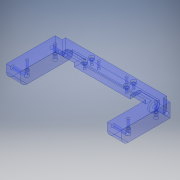
# Autodesk Inventor part: ElevBase
Saved by Autodesk Inventor 2019 (Build 230136000, 136)
## iProperties
Created: 2019-10-03
Part Number: ElevBase
Material: Generic
Document SubType Name: Modeling
Designer: james
Density: 1 g/cm^3
Appearance: Clear - Blue
Author: james
Autodesk Inventor part; units mm, degrees
ref_plane "YZ Plane" through (0, 0, 0) normal (1, 0, 0) x (0, 1, 0)
ref_plane "XZ Plane" through (0, 0, 0) normal (0, 1, 0) x (-1, 0, 0)
ref_plane "XY Plane" through (0, 0, 0) normal (0, 0, 1) x (1, 0, 0)
sketch "Sketch1" plane through (0, 0, 0) normal (0, 1, 0) x (-1, 0, 0)
  line L0 (153.7387, 43.057) -> (128.3387, 43.057)
  line L1 (128.3387, 43.057) -> (128.3387, -26.793)
  line L2 (128.3387, -26.793) -> (-30.4113, -26.793)
  line L3 (-30.4113, -26.793) -> (-30.4113, 43.057)
  line L4 (-30.4113, 43.057) -> (-55.8113, 43.057)
  line L5 (-55.8113, 43.057) -> (-55.8113, -52.193)
  line L6 (-55.8113, -52.193) -> (153.7387, -52.193)
  line L7 (153.7387, -52.193) -> (153.7387, 43.057)
  point P0 (0, 0)
  dimension "d0" = 95.25
  dimension "d1" = 25.4
  dimension "d2" = 25.4
  dimension "d3" = 158.75
  dimension "d4" = 25.4
  constraints: 16 end point, 6 perpendicular, 3 point on line, 1 horizontal
  measures "d0" distance of L6.end L0.start
  measures "d1" distance between parallel lines of L1 L7
  measures "d2" distance between parallel lines of L5 L3
  measures "d3" distance between parallel lines of L1 L3
  measures "d4" distance between parallel lines of L2 L6
extrude "Extrusion1" add sketch "Sketch1" along normal blind 25.4
sketch "Sketch2" plane through (55.8113, 0, 43.057) normal (1, 0, 0) x (0, 0, -1)
  line L0 (0, 0) -> (0, 25.4) projected
  line L1 (0, 0) -> (95.25, 0) projected
  point P0 (43.057, 0)
  point P1 (10.16, 15.24)
  dimension "d7" = 10.16
  dimension "d8" = 15.24
  measures "d7" distance from line of L0 point (10.16, 15.24)
  measures "d8" distance from line of L1 point (10.16, 15.24)
hole "Hole1" at (55.8113, 15.24, 32.897) direction (-1, 0, 0) diameter 6.477 end through all
fillet "Fillet2" radius 12.7 2 edges at (-141.0387, 0, 43.057) (43.1113, 0, 43.057)
sketch "Sketch3" plane through (0, 25.4, 0) normal (0, 1, 0) x (1, 0, 0)
  line L0 (-153.7387, 52.193) -> (-153.7387, -43.057) projected
  line L1 (55.8113, 52.193) -> (-153.7387, 52.193) projected
  line L2 (-128.3387, 26.793) -> (30.4113, 26.793) projected
  line L3 (55.8113, -43.057) -> (55.8113, 52.193) projected
  point P0 (0, 0)
  point P1 (-87.0637, 45.843)
  point P2 (-87.0637, 33.143)
  point P3 (-10.8637, 45.843)
  point P4 (-10.8637, 33.143)
  dimension "d19" = 66.675
  dimension "d20" = 6.35
  dimension "d21" = 0
  dimension "d22" = 6.35
  dimension "d23" = 0
  dimension "d24" = 6.35
  dimension "d25" = 6.35
  dimension "d26" = 66.675
  dimension "d64" = 76.2
  measures "d19" distance from line of L0 point (-87.064, 45.843)
  measures "d20" distance from line of L1 point (-87.064, 45.843)
  measures "d21" horizontal distance of point (-87.064, 45.843) point (-87.064, 33.143)
  measures "d22" distance from line of L2 point (-87.064, 33.143)
  measures "d23" horizontal distance of point (-10.864, 33.143) point (-10.864, 45.843)
  measures "d24" distance from line of L1 point (-10.864, 45.843)
  measures "d25" distance from line of L2 point (-10.864, 33.143)
  measures "d26" distance from line of L3 point (-10.864, 33.143)
  measures "d64" distance of point (-10.864, 45.843) point (-87.064, 45.843)
hole "Hole2" at (-87.0637, 25.4, -45.843) at (-87.0637, 25.4, -33.143) at (-10.8637, 25.4, -45.843) at (-10.8637, 25.4, -33.143) direction (0, -1, 0) diameter 4.4958 end through all counterbore diameter 7.9502 counterbore depth 4.1656 clearance for "Socket Head Cap Screw" size "#8" standard "Ansi Unified Screw Threads"
sketch "Sketch5" plane through (0, 0, 0) normal (0, -1, 0) x (1, 0, 0)
  line L0 (55.8113, -52.193) -> (-153.7387, -52.193) projected
  line L1 (55.8113, 43.057) -> (55.8113, -52.193) projected
  line L2 (-153.7387, -52.193) -> (-153.7387, 43.057) projected
  point P0 (0, 0)
  point P1 (-141.0387, -33.143)
  point P2 (-141.0387, 17.657)
  point P3 (43.1113, -33.143)
  point P4 (43.1113, 17.657)
  dimension "d34" = 19.05
  dimension "d35" = 12.7
  dimension "d36" = 12.7
  dimension "d37" = 50.8
  dimension "d38" = 12.7
  dimension "d39" = 19.05
  dimension "d40" = 12.7
  dimension "d41" = 50.8
  measures "d34" distance from line of L0 point (43.111, -33.143)
  measures "d35" distance from line of L1 point (43.111, -33.143)
  measures "d36" distance from line of L1 point (43.111, 17.657)
  measures "d37" distance of point (43.111, 17.657) point (43.111, -33.143)
  measures "d38" distance from line of L2 point (-141.039, -33.143)
  measures "d39" distance from line of L0 point (-141.039, -33.143)
  measures "d40" distance from line of L2 point (-141.039, 17.657)
  measures "d41" distance of point (-141.039, -33.143) point (-141.039, 17.657)
hole "Hole3" at (-141.0387, 0, -33.143) at (-141.0387, 0, 17.657) at (43.1113, 0, -33.143) at (43.1113, 0, 17.657) direction (0, 1, 0) diameter 4.4958 end through all clearance for "Socket Head Cap Screw" size "#8" standard "Ansi Unified Screw Threads"
sketch "Sketch6" plane through (0, 0, 0) normal (0, -1, 0) x (1, 0, 0)
  circle A0 centre (43.1113, -33.143) radius 2.2479 projected
  circle A1 centre (43.1113, 17.657) radius 2.2479 projected
  circle A2 centre (-141.0387, 17.657) radius 2.2479 projected
  circle A3 centre (-141.0387, -33.143) radius 2.2479 projected
  circle A4 centre (-141.0387, -33.143) radius 3.3734
  circle A5 centre (43.1113, -33.143) radius 3.3734
  circle A6 centre (43.1113, 17.657) radius 3.3734
  circle A7 centre (-141.0387, 17.657) radius 3.3734
  point P0 (0, 0)
  dimension "d49" = 6.7469
  dimension "d50" = 6.7469
  dimension "d51" = 6.7469
  dimension "d52" = 6.7469
  constraints: 4 centre point, 4 coincident
  measures "d49" diameter of A4
  measures "d50" diameter of A5
  measures "d51" diameter of A6
  measures "d52" diameter of A7
extrude "Extrusion2" cut sketch "Sketch6" against normal blind 9.525 contours A0 | A1 | A2 | A3 | A4 | A5 | A6 | A7
sketch "Sketch7" plane through (55.8113, 0, -52.193) normal (1, 0, 0) x (0, 0, -1)
  line L0 (0, 0) -> (0, 25.4) projected
  line L1 (-95.25, 25.4) -> (0, 25.4) projected
  point P0 (-52.193, 0)
  point P1 (-12.7, 10.16)
  dimension "d55" = 12.7
  dimension "d56" = 15.24
  measures "d55" distance from line of L0 point (-12.7, 10.16)
  measures "d56" distance from line of L1 point (-12.7, 10.16)
hole "Hole4" at (55.8113, 10.16, -39.493) direction (-1, 0, 0) diameter 6.477 end through all
sketch "Sketch8" plane through (0, 0, 0) normal (0, -1, 0) x (1, 0, 0)
  line L0 (1.8363, -26.793) -> (30.4113, -26.793)
  line L1 (30.4113, -26.793) -> (30.4113, -52.193)
  line L2 (30.4113, -52.193) -> (1.8363, -52.193)
  line L3 (1.8363, -52.193) -> (1.8363, -26.793)
  line L4 (30.4113, -26.793) -> (30.4113, 30.357) projected
  line L5 (55.8113, -52.193) -> (-153.7387, -52.193) projected
  line L6 (-128.3387, -26.793) -> (30.4113, -26.793) projected
  point P0 (0, 0)
  dimension "d65" = 0
  dimension "d66" = 28.575
  dimension "d67" = 0
  dimension "d68" = 0
  constraints: 8 end point, 2 parallel, 1 horizontal, 1 perpendicular
  measures "d65" distance between parallel lines of L1 L4
  measures "d66" distance of L0.start L0.end
  measures "d67" distance between parallel lines of L5 L2
  measures "d68" distance between parallel lines of L6 L0
extrude "Extrusion3" cut sketch "Sketch8" against normal blind 12.7
sketch "Sketch9" plane through (1.8363, 0, -26.793) normal (1, 0, 0) x (0, 0, -1)
  circle A0 centre (12.7, 10.16) radius 3.2385 projected
  circle A1 centre (12.7, 10.16) radius 9.144
  point P0 (-26.793, 0)
  dimension "d71" = 18.288
  constraints: 1 centre point, 1 coincident
  measures "d71" diameter of A1
extrude "Extrusion4" cut sketch "Sketch9" along normal blind 31.75
sketch "Sketch10" plane through (0, 12.7, 0) normal (0, -1, 0) x (1, 0, 0)
  line L0 (1.8363, -18.2788) -> (30.4113, -18.2788)
  line L1 (30.4113, -18.2788) -> (30.4113, -39.493)
  line L2 (30.4113, -39.493) -> (1.8363, -39.493)
  line L3 (1.8363, -39.493) -> (1.8363, -18.2788)
  line L4 (30.4113, 30.357) -> (30.4113, 30.357) projected
  line L5 (1.8363, -52.193) -> (1.8363, -26.793) projected
  line L6 (55.8113, -36.2545) -> (55.8113, -42.7315) projected
  line L7 (30.4113, -52.193) -> (1.8363, -52.193) projected
  point P0 (0, 0)
  dimension "d74" = 0
  dimension "d75" = 0
  dimension "d76" = 12.7
  constraints: 8 end point, 2 parallel, 1 horizontal, 1 perpendicular, 1 vertical alignment
  measures "d74" horizontal extent of L1
  measures "d75" distance between parallel lines of L5 L3
  measures "d76" distance between parallel lines of L7 L2
extrude "Extrusion5" cut sketch "Sketch10" against normal blind 6.35
sketch "Sketch11" plane through (0, 0, 0) normal (0, -1, 0) x (1, 0, 0)
  line L0 (-99.7637, -10.6487) -> (-128.3387, -10.6487)
  line L1 (-128.3387, -10.6487) -> (-128.3387, -64.6766)
  line L2 (-128.3387, -64.6766) -> (-99.7637, -64.6766)
  line L3 (-99.7637, -64.6766) -> (-99.7637, -10.6487)
  line L4 (-128.3387, 30.357) -> (-128.3387, -26.793) projected
  point P0 (0, 0)
  dimension "d79" = 0
  dimension "d80" = 28.575
  constraints: 8 end point, 2 parallel, 1 horizontal, 1 perpendicular
  measures "d79" distance between parallel lines of L4 L1
  measures "d80" distance of L0.start L0.end
extrude "Extrusion6" cut sketch "Sketch11" against normal blind 12.7
sketch "Sketch12" plane through (-128.3387, 25.4, 43.057) normal (1, 0, 0) x (0, 0, -1)
  arc A0 (80.5409, -12.7) -> (84.5591, -12.7) centre (82.55, -15.24) ccw projected
  circle A1 centre (82.55, -15.24) radius 9.017
  point P0 (43.057, -25.4)
  dimension "d83" = 18.034
  constraints: 1 centre point, 1 coincident
  measures "d83" diameter of A1
extrude "Extrusion7" cut sketch "Sketch12" along normal blind 28.575
sketch "Sketch13" plane through (0, 12.7, 0) normal (0, -1, 0) x (1, 0, 0)
  line L0 (-99.7637, -38.9119) -> (-128.3387, -38.9119)
  line L1 (-128.3387, -38.9119) -> (-128.3387, -17.8628)
  line L2 (-128.3387, -17.8628) -> (-99.7637, -17.8628)
  line L3 (-99.7637, -17.8628) -> (-99.7637, -38.9119)
  line L4 (-128.3387, 30.357) -> (-128.3387, -52.193) projected
  line L5 (-99.7637, -26.793) -> (-99.7637, -52.193) projected
  point P0 (0, 0)
  dimension "d86" = 0
  dimension "d87" = 0
  constraints: 8 end point, 2 parallel, 1 horizontal, 1 perpendicular
  measures "d86" distance between parallel lines of L4 L1
  measures "d87" distance between parallel lines of L5 L3
extrude "Extrusion8" cut sketch "Sketch13" against normal blind 6.35
sketch "Sketch14" plane through (0, 0, 0) normal (0, -1, 0) x (1, 0, 0)
  line L0 (-99.7637, -26.793) -> (-99.7637, -52.193) projected
  line L1 (1.8363, -52.193) -> (-99.7637, -52.193) projected
  line L2 (1.8363, -52.193) -> (1.8363, -26.793) projected
  point P0 (0, 0)
  point P1 (-23.5637, -45.843)
  point P2 (-74.3637, -45.843)
  dimension "d90" = 25.4
  dimension "d91" = 6.35
  dimension "d92" = 6.35
  dimension "d93" = 25.4
  measures "d90" distance from line of point (-74.364, -45.843) L0
  measures "d91" distance from line of L1 point (-74.364, -45.843)
  measures "d92" distance from line of L1 point (-23.564, -45.843)
  measures "d93" distance from line of L2 point (-23.564, -45.843)
hole "Hole5" at (-23.5637, 0, -45.843) at (-74.3637, 0, -45.843) direction (0, 1, 0) diameter 4.4958 end through all clearance for "Socket Head Cap Screw" size "#8" standard "Ansi Unified Screw Threads"
sketch "Sketch15" plane through (0, 0, 0) normal (0, -1, 0) x (1, 0, 0)
  circle A0 centre (-23.5637, -45.843) radius 2.2479 projected
  circle A1 centre (-74.3637, -45.843) radius 2.2479 projected
  circle A2 centre (-23.5637, -45.843) radius 3.3734
  circle A3 centre (-74.3637, -45.843) radius 3.3734
  point P0 (0, 0)
  dimension "d101" = 6.7469
  dimension "d102" = 6.7469
  constraints: 2 centre point, 2 coincident
  measures "d101" diameter of A2
  measures "d102" diameter of A3
extrude "Extrusion9" cut sketch "Sketch15" against normal blind 9.525 contours A0 | A1 | A2 | A3
sketch "Sketch16" plane through (0, 0, 0) normal (0, -1, 0) x (1, 0, 0)
  line L0 (-185.4353, -67.0507) -> (-141.0387, -67.0507)
  line L1 (-141.0387, -67.0507) -> (-141.0387, -45.843)
  line L2 (-141.0387, -45.843) -> (-185.4353, -45.843)
  line L3 (-185.4353, -45.843) -> (-185.4353, -67.0507)
  line L4 (43.1113, -67.0507) -> (71.4866, -67.0507)
  line L5 (71.4866, -67.0507) -> (71.4866, -45.843)
  line L6 (71.4866, -45.843) -> (43.1113, -45.843)
  line L7 (43.1113, -45.843) -> (43.1113, -67.0507)
  line L8 (55.8113, 30.357) -> (55.8113, -52.193) projected
  line L9 (55.8113, -52.193) -> (30.4113, -52.193) projected
  line L10 (-153.7387, -52.193) -> (-153.7387, 30.357) projected
  line L11 (-128.3387, -52.193) -> (-153.7387, -52.193) projected
  point P0 (0, 0)
  dimension "d105" = 12.7
  dimension "d106" = 6.35
  dimension "d107" = 12.7
  dimension "d108" = 6.35
  constraints: 16 end point, 4 parallel, 2 horizontal, 2 perpendicular, 2 point on line
  measures "d105" distance between parallel lines of L8 L7
  measures "d106" distance between parallel lines of L9 L6
  measures "d107" distance between parallel lines of L10 L1
  measures "d108" distance between parallel lines of L11 L2
extrude "Extrusion10" cut sketch "Sketch16" against normal blind 50.8
fillet "Fillet4" radius 6.35 3 edges at (36.7613, 0, -52.193) (-48.9637, 0, -52.193) (-134.6887, 0, -52.193)
sketch "Sketch17" plane through (-128.3387, 25.4, -26.793) normal (0, 0, 1) x (1, 0, 0)
  line L0 (28.575, -74.5621) -> (130.175, -74.5621)
  line L1 (130.175, -74.5621) -> (130.175, -12.7)
  line L2 (130.175, -12.7) -> (28.575, -12.7)
  line L3 (28.575, -12.7) -> (28.575, -74.5621)
  line L4 (130.175, -25.4) -> (130.175, -6.35) projected
  line L5 (28.575, -6.35) -> (28.575, -25.4) projected
  line L6 (28.575, -25.4) -> (130.175, -25.4) projected
  point P0 (128.3387, -25.4)
  dimension "d112" = 0
  dimension "d113" = 0
  dimension "d114" = 12.7
  constraints: 8 end point, 2 parallel, 1 horizontal, 1 perpendicular
  measures "d112" distance between parallel lines of L4 L1
  measures "d113" distance between parallel lines of L5 L3
  measures "d114" distance between parallel lines of L6 L2
extrude "Extrusion11" cut sketch "Sketch17" against normal blind 50.8
body "Solid1"
